Autodesk Fusion 360 part; units mm, degrees
(part 2 of 2)
  line L274 (-7.0748, 14.241) -> (-7.0748, 13.859)
  line L275 (-6.4646, 13.8) -> (-6.4646, 13.9197)
  line L276 (-6.4646, 13.9197) -> (-6.6815, 13.9197)
  line L277 (-6.6815, 13.9197) -> (-6.6815, 13.976)
  line L278 (-6.6815, 13.976) -> (-6.4534, 14.3)
  line L279 (-6.4534, 14.3) -> (-6.4032, 14.3)
  line L280 (-6.4032, 14.3) -> (-6.4032, 13.976)
  line L281 (-6.4032, 13.976) -> (-6.3357, 13.976)
  line L282 (-6.3357, 13.976) -> (-6.3357, 13.9197)
  line L283 (-6.3357, 13.9197) -> (-6.4032, 13.9197)
  line L284 (-6.4032, 13.9197) -> (-6.4032, 13.8)
  line L285 (-6.4032, 13.8) -> (-6.4646, 13.8)
  line L286 (-6.4646, 13.976) -> (-6.4646, 14.2014)
  line L287 (-6.4646, 14.2014) -> (-6.6212, 13.976)
  line L288 (-6.6212, 13.976) -> (-6.4646, 13.976)
  line L289 (-4.5872, 13.8) -> (-4.5872, 14.3)
  line L290 (-4.5872, 14.3) -> (-4.415, 14.3)
  spline S315 degree 2 poles (-4.415, 14.3) (-4.3566, 14.3) (-4.3259, 14.2928) knots 0 0 0 1 1 1
  spline S316 degree 2 poles (-4.3259, 14.2928) (-4.283, 14.2829) (-4.2526, 14.257) knots 0 0 0 1 1 1
  spline S317 degree 2 poles (-4.2526, 14.257) (-4.213, 14.2236) (-4.1934, 14.1716) knots 0 0 0 1 1 1
  spline S318 degree 2 poles (-4.1934, 14.1716) (-4.1738, 14.1196) (-4.1738, 14.0527) knots 0 0 0 1 1 1
  spline S319 degree 2 poles (-4.1738, 14.0527) (-4.1738, 13.9958) (-4.1871, 13.9518) knots 0 0 0 1 1 1
  spline S320 degree 2 poles (-4.1871, 13.9518) (-4.2004, 13.9078) (-4.2212, 13.879) knots 0 0 0 1 1 1
  spline S321 degree 2 poles (-4.2212, 13.879) (-4.242, 13.8501) (-4.2668, 13.8336) knots 0 0 0 1 1 1
  spline S322 degree 2 poles (-4.2668, 13.8336) (-4.2915, 13.8171) (-4.3264, 13.8085) knots 0 0 0 1 1 1
  spline S323 degree 2 poles (-4.3264, 13.8085) (-4.3614, 13.8) (-4.4068, 13.8) knots 0 0 0 1 1 1
  line L291 (-4.4068, 13.8) -> (-4.5872, 13.8)
  line L292 (-4.521, 13.859) -> (-4.4143, 13.859)
  spline S324 degree 2 poles (-4.4143, 13.859) (-4.3648, 13.859) (-4.3367, 13.8682) knots 0 0 0 1 1 1
  spline S325 degree 2 poles (-4.3367, 13.8682) (-4.3085, 13.8774) (-4.2918, 13.8941) knots 0 0 0 1 1 1
  spline S326 degree 2 poles (-4.2918, 13.8941) (-4.2683, 13.9177) (-4.2552, 13.9574) knots 0 0 0 1 1 1
  spline S327 degree 2 poles (-4.2552, 13.9574) (-4.242, 13.9971) (-4.242, 14.0538) knots 0 0 0 1 1 1
  spline S328 degree 2 poles (-4.242, 14.0538) (-4.242, 14.1322) (-4.2678, 14.1743) knots 0 0 0 1 1 1
  spline S329 degree 2 poles (-4.2678, 14.1743) (-4.2935, 14.2164) (-4.3304, 14.2308) knots 0 0 0 1 1 1
  spline S330 degree 2 poles (-4.3304, 14.2308) (-4.357, 14.241) (-4.416, 14.241) knots 0 0 0 1 1 1
  line L293 (-4.416, 14.241) -> (-4.521, 14.241)
  line L294 (-4.521, 14.241) -> (-4.521, 13.859)
  line L295 (-4.1077, 13.931) -> (-4.0432, 13.9364)
  spline S331 degree 2 poles (-4.0432, 13.9364) (-4.036, 13.8894) (-4.0099, 13.8657) knots 0 0 0 1 1 1
  spline S332 degree 2 poles (-4.0099, 13.8657) (-3.9838, 13.842) (-3.947, 13.842) knots 0 0 0 1 1 1
  spline S333 degree 2 poles (-3.947, 13.842) (-3.9027, 13.842) (-3.872, 13.8754) knots 0 0 0 1 1 1
  spline S334 degree 2 poles (-3.872, 13.8754) (-3.8413, 13.9088) (-3.8413, 13.9641) knots 0 0 0 1 1 1
  spline S335 degree 2 poles (-3.8413, 13.9641) (-3.8413, 14.0166) (-3.8708, 14.0469) knots 0 0 0 1 1 1
  spline S336 degree 2 poles (-3.8708, 14.0469) (-3.9003, 14.0773) (-3.948, 14.0773) knots 0 0 0 1 1 1
  spline S337 degree 2 poles (-3.948, 14.0773) (-3.9777, 14.0773) (-4.0016, 14.0638) knots 0 0 0 1 1 1
  spline S338 degree 2 poles (-4.0016, 14.0638) (-4.0255, 14.0503) (-4.0391, 14.0289) knots 0 0 0 1 1 1
  line L296 (-4.0391, 14.0289) -> (-4.0967, 14.0364)
  line L297 (-4.0967, 14.0364) -> (-4.0483, 14.2932)
  line L298 (-4.0483, 14.2932) -> (-3.7997, 14.2932)
  line L299 (-3.7997, 14.2932) -> (-3.7997, 14.2345)
  line L300 (-3.7997, 14.2345) -> (-3.9992, 14.2345)
  line L301 (-3.9992, 14.2345) -> (-4.0261, 14.1001)
  spline S339 degree 2 poles (-4.0261, 14.1001) (-3.9811, 14.1315) (-3.9317, 14.1315) knots 0 0 0 1 1 1
  spline S340 degree 2 poles (-3.9317, 14.1315) (-3.8662, 14.1315) (-3.8212, 14.0862) knots 0 0 0 1 1 1
  spline S341 degree 2 poles (-3.8212, 14.0862) (-3.7761, 14.0408) (-3.7761, 13.9695) knots 0 0 0 1 1 1
  spline S342 degree 2 poles (-3.7761, 13.9695) (-3.7761, 13.9016) (-3.8157, 13.8522) knots 0 0 0 1 1 1
  spline S343 degree 2 poles (-3.8157, 13.8522) (-3.8638, 13.7915) (-3.947, 13.7915) knots 0 0 0 1 1 1
  spline S344 degree 2 poles (-3.947, 13.7915) (-4.0152, 13.7915) (-4.0584, 13.8297) knots 0 0 0 1 1 1
  spline S345 degree 2 poles (-4.0584, 13.8297) (-4.1015, 13.8679) (-4.1077, 13.931) knots 0 0 0 1 1 1
  line L302 (-2.0285, 13.8) -> (-2.0285, 14.3)
  line L303 (-2.0285, 14.3) -> (-1.8562, 14.3)
  spline S346 degree 2 poles (-1.8562, 14.3) (-1.7979, 14.3) (-1.7672, 14.2928) knots 0 0 0 1 1 1
  spline S347 degree 2 poles (-1.7672, 14.2928) (-1.7242, 14.2829) (-1.6939, 14.257) knots 0 0 0 1 1 1
  spline S348 degree 2 poles (-1.6939, 14.257) (-1.6543, 14.2236) (-1.6347, 14.1716) knots 0 0 0 1 1 1
  spline S349 degree 2 poles (-1.6347, 14.1716) (-1.6151, 14.1196) (-1.6151, 14.0527) knots 0 0 0 1 1 1
  spline S350 degree 2 poles (-1.6151, 14.0527) (-1.6151, 13.9958) (-1.6284, 13.9518) knots 0 0 0 1 1 1
  spline S351 degree 2 poles (-1.6284, 13.9518) (-1.6417, 13.9078) (-1.6625, 13.879) knots 0 0 0 1 1 1
  spline S352 degree 2 poles (-1.6625, 13.879) (-1.6833, 13.8501) (-1.708, 13.8336) knots 0 0 0 1 1 1
  spline S353 degree 2 poles (-1.708, 13.8336) (-1.7328, 13.8171) (-1.7677, 13.8085) knots 0 0 0 1 1 1
  spline S354 degree 2 poles (-1.7677, 13.8085) (-1.8027, 13.8) (-1.8481, 13.8) knots 0 0 0 1 1 1
  line L304 (-1.8481, 13.8) -> (-2.0285, 13.8)
  line L305 (-1.9623, 13.859) -> (-1.8556, 13.859)
  spline S355 degree 2 poles (-1.8556, 13.859) (-1.8061, 13.859) (-1.778, 13.8682) knots 0 0 0 1 1 1
  spline S356 degree 2 poles (-1.778, 13.8682) (-1.7498, 13.8774) (-1.7331, 13.8941) knots 0 0 0 1 1 1
  spline S357 degree 2 poles (-1.7331, 13.8941) (-1.7096, 13.9177) (-1.6965, 13.9574) knots 0 0 0 1 1 1
  spline S358 degree 2 poles (-1.6965, 13.9574) (-1.6833, 13.9971) (-1.6833, 14.0538) knots 0 0 0 1 1 1
  spline S359 degree 2 poles (-1.6833, 14.0538) (-1.6833, 14.1322) (-1.7091, 14.1743) knots 0 0 0 1 1 1
  spline S360 degree 2 poles (-1.7091, 14.1743) (-1.7348, 14.2164) (-1.7717, 14.2308) knots 0 0 0 1 1 1
  spline S361 degree 2 poles (-1.7717, 14.2308) (-1.7983, 14.241) (-1.8573, 14.241) knots 0 0 0 1 1 1
  line L306 (-1.8573, 14.241) -> (-1.9623, 14.241)
  line L307 (-1.9623, 14.241) -> (-1.9623, 13.859)
  line L308 (-1.2304, 14.1776) -> (-1.2914, 14.1728)
  spline S362 degree 2 poles (-1.2914, 14.1728) (-1.2996, 14.2089) (-1.3146, 14.2253) knots 0 0 0 1 1 1
  spline S363 degree 2 poles (-1.3146, 14.2253) (-1.3395, 14.2516) (-1.376, 14.2516) knots 0 0 0 1 1 1
  spline S364 degree 2 poles (-1.376, 14.2516) (-1.4054, 14.2516) (-1.4275, 14.2352) knots 0 0 0 1 1 1
  spline S365 degree 2 poles (-1.4275, 14.2352) (-1.4565, 14.2141) (-1.4732, 14.1735) knots 0 0 0 1 1 1
  spline S366 degree 2 poles (-1.4732, 14.1735) (-1.4899, 14.1329) (-1.4906, 14.0578) knots 0 0 0 1 1 1
  spline S367 degree 2 poles (-1.4906, 14.0578) (-1.4685, 14.0916) (-1.4364, 14.108) knots 0 0 0 1 1 1
  spline S368 degree 2 poles (-1.4364, 14.108) (-1.4043, 14.1244) (-1.3692, 14.1244) knots 0 0 0 1 1 1
  spline S369 degree 2 poles (-1.3692, 14.1244) (-1.3078, 14.1244) (-1.2647, 14.0792) knots 0 0 0 1 1 1
  spline S370 degree 2 poles (-1.2647, 14.0792) (-1.2215, 14.034) (-1.2215, 13.9623) knots 0 0 0 1 1 1
  spline S371 degree 2 poles (-1.2215, 13.9623) (-1.2215, 13.9153) (-1.2418, 13.8749) knots 0 0 0 1 1 1
  spline S372 degree 2 poles (-1.2418, 13.8749) (-1.2621, 13.8344) (-1.2976, 13.813) knots 0 0 0 1 1 1
  spline S373 degree 2 poles (-1.2976, 13.813) (-1.333, 13.7915) (-1.3781, 13.7915) knots 0 0 0 1 1 1
  spline S374 degree 2 poles (-1.3781, 13.7915) (-1.4548, 13.7915) (-1.5032, 13.8479) knots 0 0 0 1 1 1
  spline S375 degree 2 poles (-1.5032, 13.8479) (-1.5517, 13.9044) (-1.5517, 14.034) knots 0 0 0 1 1 1
  spline S376 degree 2 poles (-1.5517, 14.034) (-1.5517, 14.1789) (-1.4981, 14.2447) knots 0 0 0 1 1 1
  spline S377 degree 2 poles (-1.4981, 14.2447) (-1.4514, 14.302) (-1.3723, 14.302) knots 0 0 0 1 1 1
  spline S378 degree 2 poles (-1.3723, 14.302) (-1.3133, 14.302) (-1.2756, 14.269) knots 0 0 0 1 1 1
  spline S379 degree 2 poles (-1.2756, 14.269) (-1.2379, 14.2359) (-1.2304, 14.1776) knots 0 0 0 1 1 1
  spline S380 degree 2 poles (-1.4811, 13.962) (-1.4811, 13.9303) (-1.4676, 13.9013) knots 0 0 0 1 1 1
  spline S381 degree 2 poles (-1.4676, 13.9013) (-1.4541, 13.8723) (-1.4299, 13.8571) knots 0 0 0 1 1 1
  spline S382 degree 2 poles (-1.4299, 13.8571) (-1.4057, 13.842) (-1.3791, 13.842) knots 0 0 0 1 1 1
  spline S383 degree 2 poles (-1.3791, 13.842) (-1.3402, 13.842) (-1.3122, 13.8733) knots 0 0 0 1 1 1
  spline S384 degree 2 poles (-1.3122, 13.8733) (-1.2843, 13.9047) (-1.2843, 13.9586) knots 0 0 0 1 1 1
  spline S385 degree 2 poles (-1.2843, 13.9586) (-1.2843, 14.0104) (-1.3119, 14.0403) knots 0 0 0 1 1 1
  spline S386 degree 2 poles (-1.3119, 14.0403) (-1.3395, 14.0701) (-1.3815, 14.0701) knots 0 0 0 1 1 1
  spline S387 degree 2 poles (-1.3815, 14.0701) (-1.4231, 14.0701) (-1.4521, 14.0403) knots 0 0 0 1 1 1
  spline S388 degree 2 poles (-1.4521, 14.0403) (-1.4811, 14.0104) (-1.4811, 13.962) knots 0 0 0 1 1 1
  line L309 (0.528, 13.8) -> (0.528, 14.3)
  line L310 (0.528, 14.3) -> (0.7003, 14.3)
  spline S389 degree 2 poles (0.7003, 14.3) (0.7586, 14.3) (0.7893, 14.2928) knots 0 0 0 1 1 1
  spline S390 degree 2 poles (0.7893, 14.2928) (0.8322, 14.2829) (0.8626, 14.257) knots 0 0 0 1 1 1
  spline S391 degree 2 poles (0.8626, 14.257) (0.9022, 14.2236) (0.9218, 14.1716) knots 0 0 0 1 1 1
  spline S392 degree 2 poles (0.9218, 14.1716) (0.9414, 14.1196) (0.9414, 14.0527) knots 0 0 0 1 1 1
  spline S393 degree 2 poles (0.9414, 14.0527) (0.9414, 13.9958) (0.9281, 13.9518) knots 0 0 0 1 1 1
  spline S394 degree 2 poles (0.9281, 13.9518) (0.9148, 13.9078) (0.894, 13.879) knots 0 0 0 1 1 1
  spline S395 degree 2 poles (0.894, 13.879) (0.8732, 13.8501) (0.8484, 13.8336) knots 0 0 0 1 1 1
  spline S396 degree 2 poles (0.8484, 13.8336) (0.8237, 13.8171) (0.7888, 13.8085) knots 0 0 0 1 1 1
  spline S397 degree 2 poles (0.7888, 13.8085) (0.7538, 13.8) (0.7084, 13.8) knots 0 0 0 1 1 1
  line L311 (0.7084, 13.8) -> (0.528, 13.8)
  line L312 (0.5942, 13.859) -> (0.7009, 13.859)
  spline S398 degree 2 poles (0.7009, 13.859) (0.7504, 13.859) (0.7785, 13.8682) knots 0 0 0 1 1 1
  spline S399 degree 2 poles (0.7785, 13.8682) (0.8067, 13.8774) (0.8234, 13.8941) knots 0 0 0 1 1 1
  spline S400 degree 2 poles (0.8234, 13.8941) (0.8469, 13.9177) (0.86, 13.9574) knots 0 0 0 1 1 1
  spline S401 degree 2 poles (0.86, 13.9574) (0.8732, 13.9971) (0.8732, 14.0538) knots 0 0 0 1 1 1
  spline S402 degree 2 poles (0.8732, 14.0538) (0.8732, 14.1322) (0.8474, 14.1743) knots 0 0 0 1 1 1
  spline S403 degree 2 poles (0.8474, 14.1743) (0.8217, 14.2164) (0.7848, 14.2308) knots 0 0 0 1 1 1
  spline S404 degree 2 poles (0.7848, 14.2308) (0.7582, 14.241) (0.6992, 14.241) knots 0 0 0 1 1 1
  line L313 (0.6992, 14.241) -> (0.5942, 14.241)
  line L314 (0.5942, 14.241) -> (0.5942, 13.859)
  line L315 (1.0116, 14.2345) -> (1.0116, 14.2935)
  line L316 (1.0116, 14.2935) -> (1.3353, 14.2935)
  line L317 (1.3353, 14.2935) -> (1.3353, 14.2458)
  spline S405 degree 2 poles (1.3353, 14.2458) (1.2876, 14.195) (1.2407, 14.1107) knots 0 0 0 1 1 1
  spline S406 degree 2 poles (1.2407, 14.1107) (1.1938, 14.0265) (1.1682, 13.9374) knots 0 0 0 1 1 1
  spline S407 degree 2 poles (1.1682, 13.9374) (1.1498, 13.8747) (1.1447, 13.8) knots 0 0 0 1 1 1
  line L318 (1.1447, 13.8) -> (1.0816, 13.8)
  spline S408 degree 2 poles (1.0816, 13.8) (1.0826, 13.859) (1.1048, 13.9426) knots 0 0 0 1 1 1
  spline S409 degree 2 poles (1.1048, 13.9426) (1.1269, 14.0261) (1.1684, 14.1037) knots 0 0 0 1 1 1
  spline S410 degree 2 poles (1.1684, 14.1037) (1.2098, 14.1813) (1.2565, 14.2345) knots 0 0 0 1 1 1
  line L319 (1.2565, 14.2345) -> (1.0116, 14.2345)
  line L320 (2.8533, 13.8) -> (2.8533, 14.3)
  line L321 (2.8533, 14.3) -> (3.0409, 14.3)
  spline S411 degree 2 poles (3.0409, 14.3) (3.0982, 14.3) (3.1328, 14.2848) knots 0 0 0 1 1 1
  spline S412 degree 2 poles (3.1328, 14.2848) (3.1674, 14.2696) (3.187, 14.2381) knots 0 0 0 1 1 1
  spline S413 degree 2 poles (3.187, 14.2381) (3.2066, 14.2065) (3.2066, 14.1721) knots 0 0 0 1 1 1
  spline S414 degree 2 poles (3.2066, 14.1721) (3.2066, 14.14) (3.1892, 14.1117) knots 0 0 0 1 1 1
  spline S415 degree 2 poles (3.1892, 14.1117) (3.1718, 14.0834) (3.1367, 14.066) knots 0 0 0 1 1 1
  spline S416 degree 2 poles (3.1367, 14.066) (3.1821, 14.0527) (3.2064, 14.0207) knots 0 0 0 1 1 1
  spline S417 degree 2 poles (3.2064, 14.0207) (3.2308, 13.9886) (3.2308, 13.945) knots 0 0 0 1 1 1
  spline S418 degree 2 poles (3.2308, 13.945) (3.2308, 13.9098) (3.216, 13.8796) knots 0 0 0 1 1 1
  spline S419 degree 2 poles (3.216, 13.8796) (3.2012, 13.8495) (3.1793, 13.8331) knots 0 0 0 1 1 1
  spline S420 degree 2 poles (3.1793, 13.8331) (3.1575, 13.8167) (3.1246, 13.8084) knots 0 0 0 1 1 1
  spline S421 degree 2 poles (3.1246, 13.8084) (3.0917, 13.8) (3.0439, 13.8) knots 0 0 0 1 1 1
  line L322 (3.0439, 13.8) -> (2.8533, 13.8)
  line L323 (2.9194, 14.0899) -> (3.0276, 14.0899)
  spline S422 degree 2 poles (3.0276, 14.0899) (3.0716, 14.0899) (3.0907, 14.0957) knots 0 0 0 1 1 1
  spline S423 degree 2 poles (3.0907, 14.0957) (3.1159, 14.1032) (3.1287, 14.1206) knots 0 0 0 1 1 1
  spline S424 degree 2 poles (3.1287, 14.1206) (3.1415, 14.138) (3.1415, 14.1643) knots 0 0 0 1 1 1
  spline S425 degree 2 poles (3.1415, 14.1643) (3.1415, 14.1892) (3.1295, 14.2081) knots 0 0 0 1 1 1
  spline S426 degree 2 poles (3.1295, 14.2081) (3.1176, 14.227) (3.0954, 14.234) knots 0 0 0 1 1 1
  spline S427 degree 2 poles (3.0954, 14.234) (3.0733, 14.241) (3.0194, 14.241) knots 0 0 0 1 1 1
  line L324 (3.0194, 14.241) -> (2.9194, 14.241)
  line L325 (2.9194, 14.241) -> (2.9194, 14.0899)
  line L326 (2.9194, 13.859) -> (3.0439, 13.859)
  spline S428 degree 2 poles (3.0439, 13.859) (3.076, 13.859) (3.0889, 13.8614) knots 0 0 0 1 1 1
  spline S429 degree 2 poles (3.0889, 13.8614) (3.1118, 13.8655) (3.1271, 13.875) knots 0 0 0 1 1 1
  spline S430 degree 2 poles (3.1271, 13.875) (3.1425, 13.8846) (3.1524, 13.9028) knots 0 0 0 1 1 1
  spline S431 degree 2 poles (3.1524, 13.9028) (3.1623, 13.9211) (3.1623, 13.945) knots 0 0 0 1 1 1
  spline S432 degree 2 poles (3.1623, 13.945) (3.1623, 13.9729) (3.148, 13.9936) knots 0 0 0 1 1 1
  spline S433 degree 2 poles (3.148, 13.9936) (3.1336, 14.0142) (3.1082, 14.0225) knots 0 0 0 1 1 1
  spline S434 degree 2 poles (3.1082, 14.0225) (3.0828, 14.0309) (3.0351, 14.0309) knots 0 0 0 1 1 1
  line L327 (3.0351, 14.0309) -> (2.9194, 14.0309)
  line L328 (2.9194, 14.0309) -> (2.9194, 13.859)
  line L329 (3.3192, 13.8) -> (3.3192, 14.3)
  line L330 (3.3192, 14.3) -> (3.3853, 14.3)
  line L331 (3.3853, 14.3) -> (3.3853, 13.859)
  line L332 (3.3853, 13.859) -> (3.6316, 13.859)
  line L333 (3.6316, 13.859) -> (3.6316, 13.8)
  line L334 (3.6316, 13.8) -> (3.3192, 13.8)
  line L335 (3.6555, 13.8) -> (3.8475, 14.3)
  line L336 (3.8475, 14.3) -> (3.9188, 14.3)
  line L337 (3.9188, 14.3) -> (4.1234, 13.8)
  line L338 (4.1234, 13.8) -> (4.048, 13.8)
  line L339 (4.048, 13.8) -> (3.9897, 13.9514)
  line L340 (3.9897, 13.9514) -> (3.7806, 13.9514)
  line L341 (3.7806, 13.9514) -> (3.7257, 13.8)
  line L342 (3.7257, 13.8) -> (3.6555, 13.8)
  line L343 (3.7997, 14.0053) -> (3.9692, 14.0053)
  line L344 (3.9692, 14.0053) -> (3.9171, 14.1438)
  spline S435 degree 2 poles (3.9171, 14.1438) (3.8932, 14.2069) (3.8816, 14.2475) knots 0 0 0 1 1 1
  spline S436 degree 2 poles (3.8816, 14.2475) (3.872, 14.1994) (3.8546, 14.152) knots 0 0 0 1 1 1
  line L345 (3.8546, 14.152) -> (3.7997, 14.0053)
  line L346 (5.4111, 13.8) -> (5.4111, 14.3)
  line L347 (5.4111, 14.3) -> (5.5987, 14.3)
  spline S437 degree 2 poles (5.5987, 14.3) (5.656, 14.3) (5.6906, 14.2848) knots 0 0 0 1 1 1
  spline S438 degree 2 poles (5.6906, 14.2848) (5.7253, 14.2696) (5.7449, 14.2381) knots 0 0 0 1 1 1
  spline S439 degree 2 poles (5.7449, 14.2381) (5.7645, 14.2065) (5.7645, 14.1721) knots 0 0 0 1 1 1
  spline S440 degree 2 poles (5.7645, 14.1721) (5.7645, 14.14) (5.7471, 14.1117) knots 0 0 0 1 1 1
  spline S441 degree 2 poles (5.7471, 14.1117) (5.7297, 14.0834) (5.6946, 14.066) knots 0 0 0 1 1 1
  spline S442 degree 2 poles (5.6946, 14.066) (5.7399, 14.0527) (5.7643, 14.0207) knots 0 0 0 1 1 1
  spline S443 degree 2 poles (5.7643, 14.0207) (5.7887, 13.9886) (5.7887, 13.945) knots 0 0 0 1 1 1
  spline S444 degree 2 poles (5.7887, 13.945) (5.7887, 13.9098) (5.7739, 13.8796) knots 0 0 0 1 1 1
  spline S445 degree 2 poles (5.7739, 13.8796) (5.759, 13.8495) (5.7372, 13.8331) knots 0 0 0 1 1 1
  spline S446 degree 2 poles (5.7372, 13.8331) (5.7154, 13.8167) (5.6824, 13.8084) knots 0 0 0 1 1 1
  spline S447 degree 2 poles (5.6824, 13.8084) (5.6495, 13.8) (5.6018, 13.8) knots 0 0 0 1 1 1
  line L348 (5.6018, 13.8) -> (5.4111, 13.8)
  line L349 (5.4773, 14.0899) -> (5.5854, 14.0899)
  spline S448 degree 2 poles (5.5854, 14.0899) (5.6294, 14.0899) (5.6485, 14.0957) knots 0 0 0 1 1 1
  spline S449 degree 2 poles (5.6485, 14.0957) (5.6738, 14.1032) (5.6865, 14.1206) knots 0 0 0 1 1 1
  spline S450 degree 2 poles (5.6865, 14.1206) (5.6993, 14.138) (5.6993, 14.1643) knots 0 0 0 1 1 1
  spline S451 degree 2 poles (5.6993, 14.1643) (5.6993, 14.1892) (5.6874, 14.2081) knots 0 0 0 1 1 1
  spline S452 degree 2 poles (5.6874, 14.2081) (5.6755, 14.227) (5.6533, 14.234) knots 0 0 0 1 1 1
  spline S453 degree 2 poles (5.6533, 14.234) (5.6311, 14.241) (5.5772, 14.241) knots 0 0 0 1 1 1
  line L350 (5.5772, 14.241) -> (5.4773, 14.241)
  line L351 (5.4773, 14.241) -> (5.4773, 14.0899)
  line L352 (5.4773, 13.859) -> (5.6018, 13.859)
  spline S454 degree 2 poles (5.6018, 13.859) (5.6338, 13.859) (5.6468, 13.8614) knots 0 0 0 1 1 1
  spline S455 degree 2 poles (5.6468, 13.8614) (5.6697, 13.8655) (5.685, 13.875) knots 0 0 0 1 1 1
  spline S456 degree 2 poles (5.685, 13.875) (5.7004, 13.8846) (5.7102, 13.9028) knots 0 0 0 1 1 1
  spline S457 degree 2 poles (5.7102, 13.9028) (5.7201, 13.9211) (5.7201, 13.945) knots 0 0 0 1 1 1
  spline S458 degree 2 poles (5.7201, 13.945) (5.7201, 13.9729) (5.7058, 13.9936) knots 0 0 0 1 1 1
  spline S459 degree 2 poles (5.7058, 13.9936) (5.6915, 14.0142) (5.6661, 14.0225) knots 0 0 0 1 1 1
  spline S460 degree 2 poles (5.6661, 14.0225) (5.6407, 14.0309) (5.5929, 14.0309) knots 0 0 0 1 1 1
  line L353 (5.5929, 14.0309) -> (5.4773, 14.0309)
  line L354 (5.4773, 14.0309) -> (5.4773, 13.859)
  line L355 (5.877, 13.8) -> (5.877, 14.3)
  line L356 (5.877, 14.3) -> (5.9432, 14.3)
  line L357 (5.9432, 14.3) -> (5.9432, 13.859)
  line L358 (5.9432, 13.859) -> (6.1894, 13.859)
  line L359 (6.1894, 13.859) -> (6.1894, 13.8)
  line L360 (6.1894, 13.8) -> (5.877, 13.8)
  line L361 (6.2655, 13.8) -> (6.2655, 14.3)
  line L362 (6.2655, 14.3) -> (6.3317, 14.3)
  line L363 (6.3317, 14.3) -> (6.3317, 14.052)
  line L364 (6.3317, 14.052) -> (6.58, 14.3)
  line L365 (6.58, 14.3) -> (6.6697, 14.3)
  line L366 (6.6697, 14.3) -> (6.4599, 14.0974)
  line L367 (6.4599, 14.0974) -> (6.6789, 13.8)
  line L368 (6.6789, 13.8) -> (6.5916, 13.8)
  line L369 (6.5916, 13.8) -> (6.4135, 14.0531)
  line L370 (6.4135, 14.0531) -> (6.3317, 13.9733)
  line L371 (6.3317, 13.9733) -> (6.3317, 13.8)
  line L372 (6.3317, 13.8) -> (6.2655, 13.8)
  point P0 (35.525, 0)
  point P1 (35.525, 0)
  point P2 (38.695, 0)
  point P3 (38.695, 3.54)
  point P4 (38.695, -3.54)
  dimension "d5" = 3.05
  dimension "d6" = 5.19
  dimension "d7" = 2.725
  dimension "d8" = 2.575
  dimension "d9" = 71.05
  dimension "d10" = 24.2
  dimension "d28" = 17.76
  dimension "d29" = 3.17
  dimension "d30" = 3.54
  dimension "d31" = 3.54
  dimension "d34" = 1.75
  dimension "d35" = 2.125
  dimension "d37" = 3
  dimension "d38" = 6.9
  dimension "d39" = 0.1
  dimension "d40" = 0.875
  dimension "d43" = 38.35
  dimension "d44" = 0
  dimension "d45" = 1
  dimension "d50" = 7.775
  dimension "d51" = 0.9
  dimension "d52" = 1.75
  dimension "d53" = 1.5
  dimension "d54" = 2.345
  dimension "d57" = 38.35
  dimension "d58" = 0
  constraint coincident L4.start L5.start
  constraint midpoint L2 L4.end
  constraint midpoint L1 L5.end
  constraint concentric A0 A1
  constraint symmetric L4 A0 A2
  constraint symmetric L4 A1 A3
  constraint symmetric L5 A0 A6
  constraint symmetric L5 A1 A7
  constraint symmetric L5 A2 A4
  constraint symmetric L5 A3 A5
  constraint horizontal L6
  constraint perpendicular L6 L7
  constraint parallel L6 L8
  constraint parallel L7 L9
  constraint coincident L10 L4.start
  constraint coincident L11 L4.start
  constraint horizontal L12
  constraint vertical L13
  constraint horizontal L14
  constraint vertical L15
  constraint midpoint L15 P1
  constraint midpoint L9 P1
  constraint coincident P1 P0
  constraint midpoint L13 P2
  constraint coincident L13 P3
  constraint coincident L13 P4
  constraint coincident P3 L16.start
  constraint coincident P4 L17.start
  constraint horizontal L18
  constraint vertical L19
  constraint vertical L20
  constraint perpendicular L23 L24
  constraint midpoint L22 L25.start
  constraint perpendicular L23 L25
  constraint concentric A8 A24
  constraint coincident L6 L71.end
  constraint perpendicular L6 L71
  constraint horizontal L72
  constraint vertical L73
  constraint horizontal L74
  constraint vertical L75
  measures "d5" diameter of A0
  measures "d6" diameter of A1
  measures "d7" distance of L1 A0.centre
  measures "d8" distance of L2 A0.centre
  measures "d9" distance of L6.start L6.end
  measures "d10" distance of L6.end L7.end
  measures "d28" distance of L12.start L14.end
  measures "d29" distance of L12.start L12.end
  measures "d30" distance of P2 P3
  measures "d31" distance of P2 P4
  measures "d34" distance of L18.start L18.end
  measures "d35" distance of L18.start L20.start
  measures "d37" distance of L18 L23
  measures "d38" distance of L3 L20
  measures "d39" distance of L2 L18
  measures "d40" radius of A8
  measures "d45" diameter of A24
  measures "d50" distance of L3 L71
  measures "d51" distance of L72.start L74.end
  measures "d52" distance of L73.end L74.end
  measures "d53" distance of L6 L74
  measures "d54" distance of L6.end L75
extrude "Extruir2" add sketch "Boceto2" along normal blind 6.94 contours L6 L7 L8 L9 L15
sketch "Boceto3" plane through (0, -6.94, 0) normal (0, -1, 0) x (1, 0, 0)
  line L0 (35.525, -12.1) -> (35.525, 12.1)
  line L1 (35.525, 12.1) -> (-35.525, 12.1)
  line L2 (-35.525, 12.1) -> (-35.525, -12.1)
  line L3 (-35.525, -12.1) -> (35.525, -12.1)
  line L4 (-33.35, 10.6) -> (33.35, 10.6)
  line L5 (33.35, 10.6) -> (33.35, 9.6)
  line L6 (33.35, 9.6) -> (-33.35, 9.6)
  line L7 (-33.35, 9.6) -> (-33.35, 10.6)
  line L8 (0, 0) -> (35.525, 0) construction
  line L9 (-33.35, -10.6) -> (33.35, -10.6)
  line L10 (-33.35, -9.6) -> (-33.35, -10.6)
  line L11 (33.35, -9.6) -> (-33.35, -9.6)
  line L12 (33.35, -10.6) -> (33.35, -9.6)
  line L13 (32.115, 6.855) -> (-32.115, 6.855)
  line L14 (-32.115, 6.855) -> (-32.115, -6.855)
  line L15 (-32.115, -6.855) -> (32.115, -6.855)
  line L16 (32.115, -6.855) -> (32.115, 6.855)
  line L17 (32.115, 6.855) -> (-32.115, -6.855) construction
  line L18 (-32.115, 6.855) -> (32.115, -6.855) construction
  dimension "d13" = 1
  dimension "d14" = 66.7
  dimension "d15" = 2.175
  dimension "d16" = 2.175
  dimension "d17" = 1.5
  dimension "d20" = 13.71
  dimension "d21" = 64.23
  constraint horizontal L4
  constraint vertical L5
  constraint horizontal L6
  constraint vertical L7
  constraint coincident L8.start origin
  constraint midpoint L0 L8.end
  constraint symmetric L4.start L8 L9.start
  constraint symmetric L4.end L8 L9.end
  constraint symmetric L5.end L8 L11.start
  constraint symmetric L6.end L8 L10.start
  constraint horizontal L13
  constraint perpendicular L13 L14
  constraint parallel L13 L15
  constraint parallel L14 L16
  constraint coincident L17 L8.start
  constraint coincident L18 L8.start
  measures "d13" distance of L4.start L6.end
  measures "d14" distance of L5.end L6.end
  measures "d15" distance of L2 L7
  measures "d16" distance of L0 L5
  measures "d17" distance of L1 L4
  measures "d20" distance of L13.start L15.end
  measures "d21" distance of L13.start L13.end
extrude "Extruir3" cut sketch "Boceto3" against normal blind 0.2 contours L4 L5 L6 L7 | L9 L10 L11 L12
extrude "Extruir4" cut sketch "Boceto3" against normal blind 0.25 contours L13 L14 L15 L16
extrude "Extruir5" add sketch "Boceto2" along normal blind 0.01 contours L0 A5 | L2 A3 | L0 A7 | L2 A1 | L18 L19 L20 A8 | L26 L27 A9 L28 | L29 L30 A10 L31 | L32 L33 A11 L34 | L35 L36 A12 L37 | L38 L39 A13 L40 | L41 L42 A14 L43 | L44 L45 A15 L46 | L47 L48 A16 L49 | L50 L51 A17 L52 | L53 L54 A18 L55 | L56 L57 A19 L58 | L59 L60 A20 L61 | L62 L63 A21 L64 | L65 L66 A22 L67 | L68 L69 A23 L70 picked at (-37.317, -17.6886) picked at (-37.317, 17.6886) picked at (37.393, -17.6886) picked at (37.393, 17.6886)
extrude "Extruir6" cut 4 faces at (-36.3609, 0, 15.6148) (-38.3491, 0, -15.3152) (36.3609, 0, -15.3152) (38.3491, 0, 15.6148) along direction (0, 1, 0) blind 1.61
extrude "Extruir7" add sketch "Boceto2" along normal blind 2.78 contours L9 L13 L15 L16 L17
extrude "Extruir8" cut sketch "Boceto2" against normal blind 1.61 contours A24 | A25 | A26 | A27 | A28 | A29 | A30 | A31 | A32 | A33 | A34 | A35 | A36 | A37 | A38 | A39
extrude "Extruir9" add sketch "Boceto2" along normal blind 0.01 contours L136 L137 L138 S0 S1 S2 S3 S4 S5 S6 S7 S8 S9 S10 L139 S11 S12 S13 S14 S15 S16 S17 S18 S19 S20 S21 S22 L140 L141 | L142 L143 L144 L145 L146 L147 L148 L149 L150 L151 | L152 L153 S23 S24 S25 S26 S27 S28 S29 S30 S31 L154 | L158 L159 L160 S39 S40 L161 L162 L163 L164 | L165 L166 S41 S42 S43 S44 S45 S46 S47 S48 S49 L167 | L171 L172 S57 S58 S59 S60 S61 S62 S63 S64 S65 L173 | L177 L178 L179 S73 S74 L180 L181 L182 L183 | S75 S76 S77 S78 S79 S80 S81 S82 S83 S84 S85 S86 | L184 L185 S95 S96 S97 S98 S99 S100 S101 L186 L187 L188 S102 S103 S104 S105 L189 L190 L191 | L195 S111 S112 S113 S114 S115 S116 S117 S118 S119 S120 S121 S122 S123 S124 S125 S126 S127 S128 L196 S129 S130 S131 S132 S133 S134 S135 S136 S137 S138 S139 S140 S141 S142 S143 | L197 L198 S144 S145 S146 S147 S148 S149 S150 L199 L200 L201 S151 S152 S153 S154 L202 L203 L204 | L208 L209 L210 S160 S161 L211 L212 L213 S162 S163 L214 L215 L216 L217 L218 S164 S165 L219 L220 | L221 L222 L223 L224 L225 L226 L227 L228 L229 L230 L231 L232 | L233 L234 S166 S167 S168 S169 S170 S171 S172 S173 S174 L235 | S182 S183 S184 S185 S186 S187 S188 S189 S190 S191 S192 S193 | L239 L240 S202 S203 S204 S205 S206 S207 S208 S209 S210 L241 | L245 L246 S218 S219 L247 S220 S221 L248 L249 | L250 L251 S222 S223 S224 S225 S226 S227 S228 S229 S230 L252 | L256 L257 S238 S239 S240 S241 S242 S243 S244 S245 S246 L258 S247 S248 S249 S250 S251 S252 S253 S254 S255 L259 | L260 L261 S256 S257 S258 S259 S260 S261 S262 S263 S264 L262 | L266 S272 S273 S274 S275 S276 S277 S278 L267 S279 S280 S281 S282 S283 S284 S285 L268 S286 S287 S288 S289 S290 S291 S292 S293 S294 S295 S296 S297 S298 | L269 L270 S299 S300 S301 S302 S303 S304 S305 S306 S307 L271 | L275 L276 L277 L278 L279 L280 L281 L282 L283 L284 L285 | L289 L290 S315 S316 S317 S318 S319 S320 S321 S322 S323 L291 | L295 S331 S332 S333 S334 S335 S336 S337 S338 L296 L297 L298 L299 L300 L301 S339 S340 S341 S342 S343 S344 S345 | L302 L303 S346 S347 S348 S349 S350 S351 S352 S353 S354 L304 | L308 S362 S363 S364 S365 S366 S367 S368 S369 S370 S371 S372 S373 S374 S375 S376 S377 S378 S379 | L309 L310 S389 S390 S391 S392 S393 S394 S395 S396 S397 L311 | L315 L316 L317 S405 S406 S407 L318 S408 S409 S410 L319 | L320 L321 S411 S412 S413 S414 S415 S416 S417 S418 S419 S420 S421 L322 | L329 L330 L331 L332 L333 L334 | L335 L336 L337 L338 L339 L340 L341 L342 | L346 L347 S437 S438 S439 S440 S441 S442 S443 S444 S445 S446 S447 L348 | L355 L356 L357 L358 L359 L360 | L361 L362 L363 L364 L365 L366 L367 L368 L369 L370 L371 L372
sketch "Boceto4" plane through (0, 1.61, 0) normal (0, 1, 0) x (-1, 0, 0)
  circle A0 centre (-0.9317, 15.815) radius 0.5
  circle A1 centre (9.295, 15.815) radius 0.5
  circle A2 centre (19.5217, 15.815) radius 0.5
  circle A3 centre (29.7483, 15.815) radius 0.5
  circle A4 centre (27.1917, 15.815) radius 0.5
  circle A5 centre (16.965, 15.815) radius 0.5
  circle A6 centre (6.7383, 15.815) radius 0.5
  circle A7 centre (-3.4883, 15.815) radius 0.5
  circle A8 centre (1.625, 15.815) radius 0.5
  circle A9 centre (11.8517, 15.815) radius 0.5
  circle A10 centre (22.0783, 15.815) radius 0.5
  circle A11 centre (32.305, 15.815) radius 0.5
  circle A12 centre (24.635, 15.815) radius 0.5
  circle A13 centre (14.4083, 15.815) radius 0.5
  circle A14 centre (4.1817, 15.815) radius 0.5
  circle A15 centre (-6.045, 15.815) radius 0.5
  circle A16 centre (-37.355, -15.465) radius 1.525
  circle A17 centre (37.355, 15.465) radius 1.525
  circle A18 centre (37.355, -15.465) radius 1.525
  circle A19 centre (-37.355, 15.465) radius 1.525
  line L0 (-40.08, -18.04) -> (40.08, -18.04)
  line L1 (40.08, -18.04) -> (40.08, 18.04)
  line L2 (40.08, 18.04) -> (-40.08, 18.04)
  line L3 (-40.08, 18.04) -> (-40.08, -18.04)
  circle A20 centre (-37.355, 15.465) radius 2.595
  circle A21 centre (37.355, 15.465) radius 2.595
  circle A22 centre (-37.355, -15.465) radius 2.595
  circle A23 centre (37.355, -15.465) radius 2.595
  dimension "d77" = 5.19
  dimension "d78" = 5.19
  dimension "d79" = 5.19
  dimension "d80" = 5.19
  constraint concentric A19 A20
  constraint concentric A17 A21
  constraint concentric A16 A22
  constraint concentric A18 A23
  measures "d77" diameter of A20
  measures "d78" diameter of A21
  measures "d79" diameter of A22
  measures "d80" diameter of A23
extrude "Extruir10" add sketch "Boceto4" along normal blind 0.01 contours L0 A22 | L2 A20 | L0 A23 | L2 A21 picked at (-37.317, -17.6886) picked at (-37.317, 17.6886) picked at (37.393, -17.6886) picked at (37.393, 17.6886)
sketch "Boceto5" plane through (0, 1.61, 0) normal (0, 1, 0) x (-1, 0, 0)
  circle A0 centre (-0.9317, 15.815) radius 0.5
  circle A1 centre (9.295, 15.815) radius 0.5
  circle A2 centre (19.5217, 15.815) radius 0.5
  circle A3 centre (29.7483, 15.815) radius 0.5
  circle A4 centre (27.1917, 15.815) radius 0.5
  circle A5 centre (16.965, 15.815) radius 0.5
  circle A6 centre (6.7383, 15.815) radius 0.5
  circle A7 centre (-3.4883, 15.815) radius 0.5
  circle A8 centre (1.625, 15.815) radius 0.5
  circle A9 centre (11.8517, 15.815) radius 0.5
  circle A10 centre (22.0783, 15.815) radius 0.5
  circle A11 centre (32.305, 15.815) radius 0.5
  circle A12 centre (24.635, 15.815) radius 0.5
  circle A13 centre (14.4083, 15.815) radius 0.5
  circle A14 centre (4.1817, 15.815) radius 0.5
  circle A15 centre (-6.045, 15.815) radius 0.5
  arc A16 (-37.0334, -18.04) -> (-37.6766, -18.04) centre (-37.355, -15.465) ccw
  line L0 (-37.0334, -18.04) -> (37.0334, -18.04)
  arc A17 (37.6766, -18.04) -> (37.0334, -18.04) centre (37.355, -15.465) ccw
  line L1 (37.6766, -18.04) -> (40.08, -18.04)
  line L2 (40.08, -18.04) -> (40.08, 18.04)
  line L3 (40.08, 18.04) -> (37.6766, 18.04)
  arc A18 (37.0334, 18.04) -> (37.6766, 18.04) centre (37.355, 15.465) ccw
  line L4 (37.0334, 18.04) -> (-37.0334, 18.04)
  arc A19 (-37.6766, 18.04) -> (-37.0334, 18.04) centre (-37.355, 15.465) ccw
  line L5 (-37.6766, 18.04) -> (-40.08, 18.04)
  line L6 (-40.08, 18.04) -> (-40.08, -18.04)
  line L7 (-40.08, -18.04) -> (-37.6766, -18.04)
  line L8 (31.43, 17.94) -> (33.18, 17.94)
  line L9 (33.18, 17.94) -> (33.18, 15.815)
  line L10 (31.43, 17.94) -> (31.43, 15.815)
  arc A20 (31.43, 15.815) -> (33.18, 15.815) centre (32.305, 15.815) ccw
  line L11 (28.8733, 17.94) -> (30.6233, 17.94)
  line L12 (28.8733, 17.94) -> (28.8733, 15.815)
  arc A21 (28.8733, 15.815) -> (30.6233, 15.815) centre (29.7483, 15.815) ccw
  line L13 (30.6233, 17.94) -> (30.6233, 15.815)
  line L14 (26.3167, 17.94) -> (28.0667, 17.94)
  line L15 (26.3167, 17.94) -> (26.3167, 15.815)
  arc A22 (26.3167, 15.815) -> (28.0667, 15.815) centre (27.1917, 15.815) ccw
  line L16 (28.0667, 17.94) -> (28.0667, 15.815)
  line L17 (23.76, 17.94) -> (25.51, 17.94)
  line L18 (23.76, 17.94) -> (23.76, 15.815)
  arc A23 (23.76, 15.815) -> (25.51, 15.815) centre (24.635, 15.815) ccw
  line L19 (25.51, 17.94) -> (25.51, 15.815)
  line L20 (21.2033, 17.94) -> (22.9533, 17.94)
  line L21 (21.2033, 17.94) -> (21.2033, 15.815)
  arc A24 (21.2033, 15.815) -> (22.9533, 15.815) centre (22.0783, 15.815) ccw
  line L22 (22.9533, 17.94) -> (22.9533, 15.815)
  line L23 (18.6467, 17.94) -> (20.3967, 17.94)
  line L24 (18.6467, 17.94) -> (18.6467, 15.815)
  arc A25 (18.6467, 15.815) -> (20.3967, 15.815) centre (19.5217, 15.815) ccw
  line L25 (20.3967, 17.94) -> (20.3967, 15.815)
  line L26 (16.09, 17.94) -> (17.84, 17.94)
  line L27 (16.09, 17.94) -> (16.09, 15.815)
  arc A26 (16.09, 15.815) -> (17.84, 15.815) centre (16.965, 15.815) ccw
  line L28 (17.84, 17.94) -> (17.84, 15.815)
  line L29 (13.5333, 17.94) -> (15.2833, 17.94)
  line L30 (13.5333, 17.94) -> (13.5333, 15.815)
  arc A27 (13.5333, 15.815) -> (15.2833, 15.815) centre (14.4083, 15.815) ccw
  line L31 (15.2833, 17.94) -> (15.2833, 15.815)
  line L32 (10.9767, 17.94) -> (12.7267, 17.94)
  line L33 (10.9767, 17.94) -> (10.9767, 15.815)
  arc A28 (10.9767, 15.815) -> (12.7267, 15.815) centre (11.8517, 15.815) ccw
  line L34 (12.7267, 17.94) -> (12.7267, 15.815)
  line L35 (8.42, 17.94) -> (10.17, 17.94)
  line L36 (8.42, 17.94) -> (8.42, 15.815)
  arc A29 (8.42, 15.815) -> (10.17, 15.815) centre (9.295, 15.815) ccw
  line L37 (10.17, 17.94) -> (10.17, 15.815)
  line L38 (5.8633, 17.94) -> (7.6133, 17.94)
  line L39 (5.8633, 17.94) -> (5.8633, 15.815)
  arc A30 (5.8633, 15.815) -> (7.6133, 15.815) centre (6.7383, 15.815) ccw
  line L40 (7.6133, 17.94) -> (7.6133, 15.815)
  line L41 (3.3067, 17.94) -> (5.0567, 17.94)
  line L42 (3.3067, 17.94) -> (3.3067, 15.815)
  arc A31 (3.3067, 15.815) -> (5.0567, 15.815) centre (4.1817, 15.815) ccw
  line L43 (5.0567, 17.94) -> (5.0567, 15.815)
  line L44 (0.75, 17.94) -> (2.5, 17.94)
  line L45 (0.75, 17.94) -> (0.75, 15.815)
  arc A32 (0.75, 15.815) -> (2.5, 15.815) centre (1.625, 15.815) ccw
  line L46 (2.5, 17.94) -> (2.5, 15.815)
  line L47 (-1.8067, 17.94) -> (-0.0567, 17.94)
  line L48 (-1.8067, 17.94) -> (-1.8067, 15.815)
  arc A33 (-1.8067, 15.815) -> (-0.0567, 15.815) centre (-0.9317, 15.815) ccw
  line L49 (-0.0567, 17.94) -> (-0.0567, 15.815)
  line L50 (-4.3633, 17.94) -> (-2.6133, 17.94)
  line L51 (-4.3633, 17.94) -> (-4.3633, 15.815)
  arc A34 (-4.3633, 15.815) -> (-2.6133, 15.815) centre (-3.4883, 15.815) ccw
  line L52 (-2.6133, 17.94) -> (-2.6133, 15.815)
  line L53 (-6.92, 17.94) -> (-5.17, 17.94)
  line L54 (-6.92, 17.94) -> (-6.92, 15.815)
  arc A35 (-6.92, 15.815) -> (-5.17, 15.815) centre (-6.045, 15.815) ccw
  line L55 (-5.17, 17.94) -> (-5.17, 15.815)
  dimension "d83" = 0.1
  dimension "d84" = 6.9
  dimension "d85" = 2.125
  dimension "d86" = 2.125
  dimension "d87" = 1.75
  dimension "d90" = -38.35
  dimension "d91" = 0
  constraint horizontal L8
  constraint perpendicular L8 L9
  constraint perpendicular L8 L10
  constraint concentric A11 A20
  measures "d83" distance of L4 L8
  measures "d84" distance of L2 L9
  measures "d85" distance of L8.end L9.end
  measures "d86" distance of L8.start L10.end
  measures "d87" distance of L8.start L8.end
extrude "Extruir11" add sketch "Boceto5" along normal blind 0.01 contours L8 L9 L10 A20 | L11 L12 A21 L13 | L14 L15 A22 L16 | L17 L18 A23 L19 | L20 L21 A24 L22 | L23 L24 A25 L25 | L26 L27 A26 L28 | L29 L30 A27 L31 | L32 L33 A28 L34 | L35 L36 A29 L37 | L38 L39 A30 L40 | L41 L42 A31 L43 | L44 L45 A32 L46 | L47 L48 A33 L49 | L50 L51 A34 L52 | L53 L54 A35 L55
fillet "Empalme1" radius 0.5 4 edges at (0, -6.94, 12.1) (-35.525, -6.94, 0) (0, -6.94, -12.1) (35.525, -6.94, 0)
equation "d43 = 40.1 mm - 1.75 mm"
equation "d57 = 40.1 mm - 1.75 mm"
equation "d90 = -40.1 mm + 1.75 mm"
named bodies: "Display lcd 16x2"

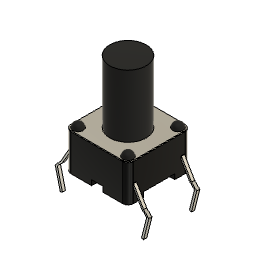
design "Push button"
Autodesk Fusion 360 part; units mm, degrees
sketch "Sketch1" plane through (0, 0, 0) normal (0, 0, 1) x (1, 0, 0)
  line L0 (0, 0) -> (6, 0)
  line L1 (0, 0) -> (0, 6)
  line L2 (0, 6) -> (6, 6)
  line L3 (6, 6) -> (6, 0)
  dimension "d1" = 6
  dimension "d2" = 6
  dimension "d3" = 6
  dimension "d4" = 6
  constraint coincident L0.start L1.start
  constraint horizontal L0
  constraint perpendicular L0 L1
  constraint perpendicular L1 L2
  constraint perpendicular L2 L3
  measures "d1" distance of L0.start L0.end
  measures "d2" distance of L0.start L1.end
  measures "d3" distance of L1.end L2.end
  measures "d4" distance of L2.end L0.end
extrude "Extrude1" add sketch "Sketch1" along normal blind 3.5 makes body 1
sketch "Sketch2" plane through (0, 0, 3.5) normal (0, 0, 1) x (-1, 0, 0)
  line L0 (0, 0) -> (-6, 0)
  line L1 (-6, 0) -> (-6, -6)
  line L2 (-6, -6) -> (0, -6)
  line L3 (0, -6) -> (0, 0)
  line L4 (0, -6) -> (-6, -6)
  line L5 (-6, -6) -> (-6, 0)
  line L6 (-6, 0) -> (0, 0)
  line L7 (0, 0) -> (0, -6)
  constraint horizontal L4
  constraint vertical L5
  constraint horizontal L6
  constraint vertical L7
  constraint coincident L0.end L1.start
  constraint coincident L2.end L3.start
extrude "Extrude1'" add sketch "Sketch2" along normal blind 0.1 separate body makes body 2 in component "Component"
fillet "Fillet1" radius 0.5 1 edges at (0, 0, 3.55) on bodies 2 in component "Component"
fillet "Fillet1'" radius 0.5 1 edges at (0, 0, 1.75) on bodies 1
fillet "Fillet2" radius 0.5 3 edges at (6, 0, 3.55) (6, 6, 3.55) (0, 6, 3.55) on bodies 2 in component "Component"
fillet "Fillet2'" radius 0.5 3 edges at (6, 0, 1.75) (6, 6, 1.75) (0, 6, 1.75) on bodies 1
sketch "Sketch3" plane through (0, 0, 3.6) normal (0, 0, 1) x (-1, 0, 0)
  arc A0 (-0.5, -6) -> (0, -5.5) centre (-0.5, -5.5) ccw
  line L0 (0, -5.5) -> (0, -0.5)
  arc A1 (0, -0.5) -> (-0.5, 0) centre (-0.5, -0.5) ccw
  line L1 (-0.5, 0) -> (-5.5, 0)
  arc A2 (-5.5, 0) -> (-6, -0.5) centre (-5.5, -0.5) ccw
  line L2 (-6, -0.5) -> (-6, -5.5)
  arc A3 (-6, -5.5) -> (-5.5, -6) centre (-5.5, -5.5) ccw
  line L3 (-5.5, -6) -> (-0.5, -6)
  circle A4 centre (-3, -3) radius 1.75
  dimension "d17" = 3.5
  measures "d17" diameter of A4
extrude "Extrude1''" add sketch "Sketch3" along normal blind 6 separate body contours A4 makes body 3 in component "Component'"
sketch "Sketch4" plane through (0, 0, 3.6) normal (0, 0, 1) x (-1, 0, 0)
  arc A0 (-0.5, -6) -> (0, -5.5) centre (-0.5, -5.5) ccw
  line L0 (0, -5.5) -> (0, -0.5)
  arc A1 (0, -0.5) -> (-0.5, 0) centre (-0.5, -0.5) ccw
  line L1 (-0.5, 0) -> (-5.5, 0)
  arc A2 (-5.5, 0) -> (-6, -0.5) centre (-5.5, -0.5) ccw
  line L2 (-6, -0.5) -> (-6, -5.5)
  arc A3 (-6, -5.5) -> (-5.5, -6) centre (-5.5, -5.5) ccw
  line L3 (-5.5, -6) -> (-0.5, -6)
  circle A4 centre (-0.6, -0.6) radius 0.5
  circle A5 centre (-5.4, -0.6) radius 0.5
  circle A6 centre (-5.4, -5.4) radius 0.5
  circle A7 centre (-0.6, -5.4) radius 0.5
  dimension "d21" = 1
  dimension "d22" = 1
  dimension "d23" = 1
  dimension "d24" = 1
  measures "d21" diameter of A4
  measures "d22" diameter of A5
  measures "d23" diameter of A6
  measures "d24" diameter of A7
extrude "Extrude1'''" add sketch "Sketch4" along normal blind 0.5 separate body contours A4 | A5 | A6 | A7 makes body 4 at (4.9025, 0.6498, 3.7667) makes body 5 at (0.1025, 0.6498, 3.7667) makes body 6 at (4.9025, 5.4498, 3.7667) makes body 7 at (0.1025, 5.4498, 3.7667) in component "Component''"
fillet "Fillet1''" radius 0.5 4 edges at (5.8662, 0.7808, 4.1) (1.0662, 0.7808, 4.1) (5.8662, 5.5808, 4.1) (1.0662, 5.5808, 4.1) on bodies 4 5 6 7 in component "Component''"
sketch "Sketch5" plane through (0, 0, 0) normal (0, 1, 0) x (1, 0, 0)
  line L0 (-0.0323, -1.6751) -> (-1, 0)
  line L1 (-1, 0) -> (-1.5, 0.5)
  line L2 (-1.5, 0.5) -> (-1, 2.5)
  line L3 (-1, 2.5) -> (-0.806, 2.4515)
  line L4 (-0.806, 2.4515) -> (-1.2938, 0.5)
  line L5 (-1.2938, 0.5) -> (-0.806, 0.0121)
  line L6 (-0.806, 0.0121) -> (0.0144, -1.4079)
  line L7 (0.0144, -1.4079) -> (0.0144, -1.6751)
  line L8 (0.0144, -1.6751) -> (-0.0323, -1.6751)
  dimension "d29" = 0.2
  constraint perpendicular L2 L3
  constraint perpendicular L3 L4
  constraint parallel L1 L5
  constraint parallel L0 L6
  constraint vertical L7
  constraint perpendicular L7 L8
  measures "d29" distance of L2.end L3.end
extrude "Extrude1''''" add sketch "Sketch5" along normal blind 0.3 separate body makes body 8 in component "Component'''"
move_body "Move1" bodies 8 to x (1, 0, 0) y (0, 1, 0) z (0, 0, 1) at (0, 0.5, 0) in component "Component'''"
copy_body "CopyPasteBodies1" bodies 8 makes body 9
move_body "Move1'" bodies 9 to x (1, 0, 0) y (0, 1, 0) z (0, 0, 1) at (0, 4.6, 0)
copy_body "CopyPasteBodies2" bodies 8 9 makes body 10 makes body 11
move_body "Move2" bodies 10 11 to x (-1, 0, 0) y (0, -1, 0) z (0, 0, 1) at (6, 5.9, 0)
sketch "Sketch6" plane through (0, 0, 0) normal (0, 0, -1) x (1, 0, 0)
  arc A0 (0, -5.5) -> (0.5, -6) centre (0.5, -5.5) ccw
  line L0 (0.5, -6) -> (5.5, -6)
  arc A1 (5.5, -6) -> (6, -5.5) centre (5.5, -5.5) ccw
  line L1 (6, -5.5) -> (6, -0.5)
  arc A2 (6, -0.5) -> (5.5, 0) centre (5.5, -0.5) ccw
  line L2 (5.5, 0) -> (0.5, 0)
  arc A3 (0.5, 0) -> (0, -0.5) centre (0.5, -0.5) ccw
  line L3 (0, -0.5) -> (0, -5.5)
  line L4 (2.5, 0) -> (3.5969, 0)
  line L5 (3.5969, 0) -> (3.5969, -6)
  line L6 (3.5969, -6) -> (2.5, -6)
  line L7 (2.5, -6) -> (2.5, 0)
  line L8 (0, -1.5) -> (1.5, -1.5)
  line L9 (1.5, -1.5) -> (1.5, -4.5)
  line L10 (1.5, -4.5) -> (0, -4.5)
  line L11 (0, -4.5) -> (0, -1.5)
  line L12 (4.5, -4.5) -> (4.5, -1.5)
  line L13 (4.5, -1.5) -> (6, -1.5)
  line L14 (6, -1.5) -> (6, -4.5)
  line L15 (6, -4.5) -> (4.5, -4.5)
  constraint horizontal L4
  constraint vertical L5
  constraint horizontal L6
  constraint vertical L7
  constraint coincident L0 L5.end
  constraint coincident L2 L4.start
  constraint horizontal L8
  constraint vertical L9
  constraint horizontal L10
  constraint vertical L11
  constraint coincident L3 L8.start
  constraint horizontal L13
  constraint vertical L14
  constraint horizontal L15
  constraint vertical L12
extrude "Extrude2" cut sketch "Sketch6" against normal blind 0.5 contours L3 L8 L9 L10 L11 | L0 L2 L4 L5 L6 L7 | L1 L12 L13 L14 L15 bodies 1
component "Component" placed x (1, 0, 0) y (0, 1, 0) z (0, 0, 1) at (0, 0, 0)
component "Component'" placed x (1, 0, 0) y (0, 1, 0) z (0, 0, 1) at (0, 0, 0)
component "Component''" placed x (1, 0, 0) y (0, 1, 0) z (0, 0, 1) at (0, 0, 0)
component "Component'''" placed x (1, 0, 0) y (0, 1, 0) z (0, 0, 1) at (0, 0, 0)
